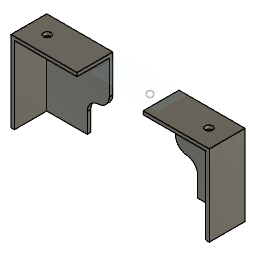
Rear Spinner And Limit Switch Bracket (Autodesk Fusion 360 design; units mm, degrees)
part number: 2026-05-02-17-09-29-765
Autodesk Fusion 360 part; units mm, degrees
sketch "Sketch1" plane through (0, 0, 0) normal (0, 0, 1) x (1, 0, 0)
  line L0 (-2.5, 0.5) -> (27.5, 0.5)
  line L1 (27.5, 0.5) -> (27.5, -1.9)
  line L2 (27.5, -1.9) -> (-2.5, -1.9)
  line L3 (-2.5, -1.9) -> (-2.5, 0.5)
  dimension "d1" = 2.4
  dimension "d2" = 30
  constraint horizontal L0
  constraint vertical L1
  constraint horizontal L2
  constraint vertical L3
  measures "d1" distance of L0.start L2.end
  measures "d2" distance of L1 L3
extrude "Extrude1" add sketch "Sketch1" along normal blind 55 makes body 1
sketch "Sketch2" plane through (0, 0.5, 0) normal (0, 1, 0) x (-1, 0, 0)
  line L0 (-27.5, 0) -> (2.5, 0)
  line L1 (2.5, 0) -> (2.5, 55)
  line L2 (2.5, 55) -> (-27.5, 55)
  line L3 (-27.5, 55) -> (-27.5, 0)
  circle A0 centre (-12.5, 40) radius 2.5
  dimension "d5" = 5
  dimension "d6" = 15
  dimension "d7" = 40
  measures "d5" diameter of A0
  measures "d6" distance of L3 A0.centre
  measures "d7" distance of L0 A0.centre
extrude "Extrude2" cut sketch "Sketch2" against normal blind 2.4 contours A0 bodies 1
sketch "Sketch3" plane through (-2.5, 0, 0) normal (-1, 0, 0) x (0, -1, 0)
  line L0 (-0.5, 0) -> (1.9, 0)
  line L1 (1.9, 0) -> (1.9, 55)
  line L2 (1.9, 55) -> (-0.5, 55)
  line L3 (-0.5, 55) -> (-0.5, 0)
  line L4 (-0.5, 55) -> (1.9, 55)
  line L5 (1.9, 55) -> (1.9, 21.6579)
  line L6 (1.9, 21.6579) -> (-0.5, 21.6579)
  line L7 (-0.5, 21.6579) -> (-0.5, 55)
  constraint horizontal L4
  constraint vertical L5
  constraint horizontal L6
  constraint vertical L7
  constraint coincident L1 L5.end
  constraint coincident L2.end L3.start
extrude "Extrude3" add sketch "Sketch3" along normal blind 15 contours L1 L2 L3 L4 L5 L6 L7 bodies 1
sketch "Sketch4" plane through (0, -1.9, 0) normal (0, -1, 0) x (1, 0, 0)
  circle A0 centre (12.5, 40) radius 2.5
  line L0 (-2.5, 0) -> (27.5, 0)
  line L1 (27.5, 0) -> (27.5, 55)
  line L2 (27.5, 55) -> (-17.5, 55)
  line L3 (-17.5, 55) -> (-17.5, 21.6579)
  line L4 (-17.5, 21.6579) -> (-2.5, 21.6579)
  line L5 (-2.5, 21.6579) -> (-2.5, 0)
  line L6 (-17.5, 55) -> (27.5, 55)
  line L7 (27.5, 55) -> (27.5, 52.6)
  line L8 (27.5, 52.6) -> (-17.5, 52.6)
  line L9 (-17.5, 52.6) -> (-17.5, 55)
  dimension "d12" = 2.4
  constraint horizontal L6
  constraint vertical L7
  constraint horizontal L8
  constraint vertical L9
  constraint coincident L2.end L3.start
  measures "d12" distance of L2.end L8.end
extrude "Extrude4" add sketch "Sketch4" along normal blind 17 contours L1 L2 L3 L6 L7 L8 L9 bodies 1
sketch "Sketch5" plane through (0, 0, 55) normal (0, 0, 1) x (-1, 0, 0)
  line L0 (-27.5, 18.9) -> (-27.5, -0.5)
  line L1 (-27.5, -0.5) -> (17.5, -0.5)
  line L2 (17.5, -0.5) -> (17.5, 18.9)
  line L3 (17.5, 18.9) -> (-27.5, 18.9)
  circle A0 centre (-15, 11.7) radius 2.5
  dimension "d15" = 5
  dimension "d16" = 12.5
  dimension "d29" = 12.2
  measures "d15" diameter of A0
  measures "d16" distance of L0 A0.centre
  measures "d29" distance of L1 A0.centre
extrude "Extrude5" cut sketch "Sketch5" against normal blind 2.4 contours A0 bodies 1
fillet "Fillet1" radius 8 1 edges at (-2.5, -0.7, 21.6579) on bodies 1
fillet "Fillet2" radius 8 1 edges at (-17.5, -0.7, 21.6579) on bodies 1
sketch "Sketch6" plane through (0, 0, 52.6) normal (0, 0, -1) x (1, 0, 0)
  circle A0 centre (15, 11.7) radius 2.5
  line L0 (-17.5, 1.9) -> (27.5, 1.9)
  line L1 (27.5, 1.9) -> (27.5, 18.9)
  line L2 (27.5, 18.9) -> (-17.5, 18.9)
  line L3 (-17.5, 18.9) -> (-17.5, 1.9)
  line L4 (27.5, 18.9) -> (25.1, 18.9)
  line L5 (25.1, 18.9) -> (25.1, 1.9)
  line L6 (25.1, 1.9) -> (27.5, 1.9)
  line L7 (27.5, 1.9) -> (27.5, 18.9)
  dimension "d24" = 2.4
  constraint horizontal L4
  constraint vertical L5
  constraint horizontal L6
  constraint vertical L7
  constraint coincident L0 L5.end
  constraint coincident L1.end L2.start
  measures "d24" distance of L5 L7
extrude "Extrude6" add sketch "Sketch6" along normal blind 52.6 contours L0 L1 L2 L4 L5 L6 L7 bodies 1
extrude "Extrude7" add 1 faces at (26.7, -18.9, 35.8667) along direction (0, -1, 0) blind 5 on bodies 1 bodies 1
mirror "Mirror1" [no effect]
move_body "Move4" bodies 1 to x (1, 0, 0) y (0, 1, 0) z (0, 0, 1) at (40, 0, 0)
mirror "Mirror2" about plane through (0, 0, 0) normal (1, 0, 0) of bodies 1 makes body 2
